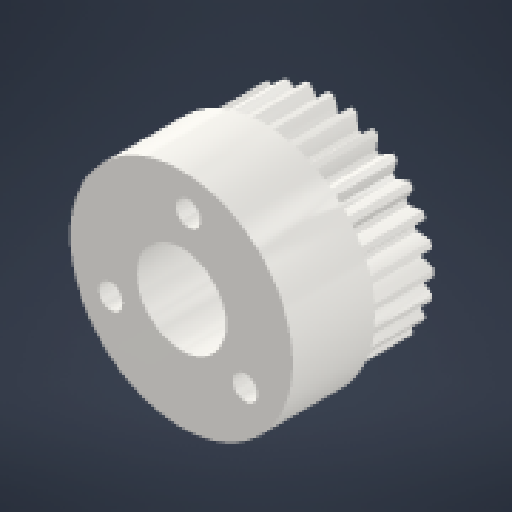
# Autodesk Inventor part: Spur Gear2
Saved by Autodesk Inventor 2025 (Build 290162000, 162)
## iProperties
CustomPartVersion: 1
Created: 2024-04-16
Part Number: Spur Gear2
Material: Steel
Document SubType Name: Modeling
Designer: sicia
Categories: <?xml version="1.0" encoding="UTF-16"?> <MemberInstance><Categories><FamilyTemplate><FamilyTemplateParameter ValueType="xs:double" Id="1" ObjectReferenceKey="da_z" ObjectType="kUserParameterObject"/><FamilyTemplateParameter ValueType="xs:double" Id="2" ObjectReferenceKey="da_b" ObjectType="kUserParameterObject"/><FamilyTemplateParameter ValueType="xs:double" Id="3" ObjectReferenceKey="da_beta" ObjectType="kUserParameterObject"/><FamilyTemplateParameter ValueType="xs:double" Id="4" ObjectReferenceKey="da_da" ObjectType="kUserParameterObject"/><FamilyTemplateParameter ValueType="xs:double" Id="5" ObjectReferenceKey="da_aw" ObjectType="kUserParameterObject"/><FamilyTemplateParameter ValueType="xs:string" Id="6" ObjectReferenceKey="EAIAABAAAACIAQAAAAAAAIAAAAAAAAAA" ObjectType="83910656" SubObjectId="SurfaceGeometry"/></FamilyTemplate><ParamToTemplateMap><ParamToTemplate CategoryParameter="//CategoryParameter[@InternalName='046C89C9-8512-4d59-83FE-43B91F4F132A']" TemplateParameter="1"/><ParamToTemplate CategoryParameter="//CategoryParameter[@InternalName='2552DF32-E462-4b46-AEBF-C6C7768E72AC']" TemplateParameter="2"/><ParamToTemplate CategoryParameter="//CategoryParameter[@InternalName='C9EE641D-15FC-4fae-A226-E94C4372FDD7']" TemplateParameter="3"/><ParamToTemplate><ParamToTemplate CategoryParameter="//CategoryParameter[@InternalName='00B6519A-459B-49c7-AD84-2E56D39A5744']" ConstantValue="0.770775"/></ParamToTemplate><ParamToTemplate><ParamToTemplate CategoryParameter="//CategoryParameter[@InternalName='04B31F0E-C7A6-4894-AA32-9629BEFACF47']" ConstantValue="1.000000"/></ParamToTemplate><ParamToTemplate><ParamToTemplate CategoryParameter="//CategoryParameter[@InternalName='43CBEC2E-7847-49e7-A936-2F7889FCB2D9']" ConstantValue="0.250000"/></ParamToTemplate><ParamToTemplate><ParamToTemplate CategoryParameter="//CategoryParameter[@InternalName='B1EFC894-105D-4ebd-86BF-FA20ED196853']" ConstantValue="0.333500"/></ParamToTemplate><ParamToTemplate><ParamToTemplate CategoryParameter="//CategoryParameter[@InternalName='51175063-3D10-4879-93E8-6246FE8B403D']" ConstantValue="2060000000.000000"/></ParamToTemplate><ParamToTemplate><ParamToTemplate CategoryParameter="//CategoryParameter[@InternalName='A3A52E27-4454-46a9-B0BD-C932399B70AF']" ConstantValue="0.300000"/></ParamToTemplate><ParamToTemplate><ParamToTemplate CategoryParameter="//CategoryParameter[@InternalName='91B76062-C214-41d9-B1B9-14D2AB99603D']" ConstantValue="0.150000"/></ParamToTemplate><ParamToTemplate><ParamToTemplate CategoryParameter="//CategoryParameter[@InternalName='374E806E-8B8A-4dda-A9AA-1039D6500AD2']" ConstantValue="6.666667"/></ParamToTemplate><ParamToTemplate><ParamToTemplate CategoryParameter="//CategoryParameter[@InternalName='2D373A89-B862-43d6-8D0B-0CBF12AB9F6C']" ConstantValue="0.349066"/></ParamToTemplate><ParamToTemplate CategoryParameter="//CategoryParameter[@InternalName='37777632-D6A2-4fac-9D53-DB8ACD95C989']" TemplateParameter="4"/><ParamToTemplate CategoryParameter="//CategoryParameter[@InternalName='FD1017F1-B727-4f7e-9707-0F86F1FF9423']" TemplateParameter="5"/><ParamToTemplate><ParamToTemplate CategoryParameter="//CategoryParameter[@InternalName='9E1B4470-B2D3-4ff1-B813-535BB4CDF51A']" ConstantValue="3520000.000000"/></ParamToTemplate><ParamToTemplate><ParamToTemplate CategoryParameter="//CategoryParameter[@InternalName='F8452263-BFF6-458c-9FB1-07C4B99E95CD']" ConstantValue="11400000.000000"/></ParamToTemplate><ParamToTemplate><ParamToTemplate CategoryParameter="//CategoryParameter[@InternalName='3E3BB259-FD49-497f-8171-6EBC954A3479']" ConstantValue="2.000000"/></ParamToTemplate><ParamToTemplate CategoryParameter="//CategoryParameter[@InternalName='27C3BAF2-7550-4e4b-AE2C-0DB134B7D9B7']" TemplateParameter="6"/></ParamToTemplateMap><Category DisplayName="Gear" InternalName="DC85795E-93AB-48d5-8EEE-5A27447B64BD" Mnemonic="Gear"><CategoryParameter DisplayName="z" InternalName="046C89C9-8512-4d59-83FE-43B91F4F132A" Mnemonic="z"/><CategoryParameter DisplayName="b" InternalName="2552DF32-E462-4b46-AEBF-C6C7768E72AC" Mnemonic="b"/><CategoryParameter DisplayName="||b|" InternalName="C9EE641D-15FC-4fae-A226-E94C4372FDD7" Mnemonic="beta"/><CategoryParameter DisplayName="x" InternalName="00B6519A-459B-49c7-AD84-2E56D39A5744" Mnemonic="x"/><CategoryParameter DisplayName="a*" InternalName="04B31F0E-C7A6-4894-AA32-9629BEFACF47" Mnemonic="a"/><CategoryParameter DisplayName="c*" InternalName="43CBEC2E-7847-49e7-A936-2F7889FCB2D9" Mnemonic="c"/><CategoryParameter DisplayName="r|.f|*" InternalName="B1EFC894-105D-4ebd-86BF-FA20ED196853" Mnemonic="rf"/><CategoryParameter DisplayName="E" InternalName="51175063-3D10-4879-93E8-6246FE8B403D" Mnemonic="E"/><CategoryParameter DisplayName="||m|" InternalName="A3A52E27-4454-46a9-B0BD-C932399B70AF" Mnemonic="mi"/><Category DisplayName="SpurGear" InternalName="26C5A22E-A91E-4dfd-A3B3-23CCAFAE1764" Mnemonic="SpurGear"><CategoryParameter DisplayName="m" InternalName="91B76062-C214-41d9-B1B9-14D2AB99603D" Mnemonic="m"/><CategoryParameter DisplayName="P" InternalName="374E806E-8B8A-4dda-A9AA-1039D6500AD2" Mnemonic="PP"/><CategoryParameter DisplayName="||a|" InternalName="2D373A89-B862-43d6-8D0B-0CBF12AB9F6C" Mnemonic="alpha"/><CategoryParameter DisplayName="d|.a|" InternalName="37777632-D6A2-4fac-9D53-DB8ACD95C989" Mnemonic="da"/><CategoryParameter DisplayName="a|.w|" InternalName="FD1017F1-B727-4f7e-9707-0F86F1FF9423" Mnemonic="aw"/><CategoryParameter DisplayName="||s||.Flim|" InternalName="9E1B4470-B2D3-4ff1-B813-535BB4CDF51A" Mnemonic="sFlim"/><CategoryParameter DisplayName="||s||.Hlim|" InternalName="F8452263-BFF6-458c-9FB1-07C4B99E95CD" Mnemonic="sHlim"/><CategoryParameter DisplayName="type" InternalName="3E3BB259-FD49-497f-8171-6EBC954A3479" Mnemonic="type"/><CategoryParameter DisplayName="PitchDiameter" InternalName="27C3BAF2-7550-4e4b-AE2C-0DB134B7D9B7" Mnemonic="IDS_PITCHDIAM"/></Category></Category></Categories></MemberInstance>
Density: 7.85 g/cm^3
Appearance: Steel
Mass: 368.86 g
Surface Area: 131.516 cm^2
Volume: 46.9885 cm^3
Author: sicia
Autodesk Inventor part; units mm, degrees
sketch "Sketch1" plane through (0, 0, 0) normal (0, 0, 1) x (1, 0, 0)
  circle A0 centre (0, 0) radius 23.3443
  dimension "d0" = 46.6886
  constraints: 1 centre point
  measures "d0" diameter of A0
extrude "Extrusion1" add sketch "Sketch1" along normal blind 10
ref_plane "Work Plane2" through (0, 0, 5) normal (0, 0, 1) x (1, 0, 0)
sketch "Sketch2" plane through (0, 0, 0) normal (0, 0, -1) x (-1, 0, 0)
  circle A0 centre (0, 0) radius 23.3443 projected
  circle A1 centre (0, 0) radius 21
  dimension "d3" = 42
  constraints: 1 centre point, 1 coincident
  measures "d3" diameter of A1
surface extrude "Pitch Diameter" sketch "Sketch2" against normal through all shown no curves A1
ref_plane "Work Plane8" through (0, 0, 0) normal (0.9937122, 0.1119645, 0) x (0, 0, 1)
ref_plane "Work Plane9" through (0, 0, 0) normal (1, 0, 0) x (0, 1, 0)
spur gear teeth "Spur Gear" teeth 28 pitch diameter 42 tip diameter 46.6886 root diameter 40.5623 face width 10 start plane through (0, 0, 0) normal (0, 0, -1) x (-1, 0, 0)
sketch "Sketch3" plane through (0, 0, 10) normal (0, 0, 1) x (1, 0, 0)
  arc A0 (-5.8309, 22.6044) -> (-6.1589, 19.3234) centre (6.5782, 19.7067) ccw projected
  arc A1 (-6.1589, 19.3234) -> (-7.2327, 18.9477) centre (0, 0) ccw projected
  arc A2 (-7.2327, 18.9477) -> (-9.5348, 21.3083) centre (-17.43, 11.3058) ccw projected
  arc A3 (-9.5348, 21.3083) -> (-10.7146, 20.7401) centre (0, 0) ccw projected
  arc A4 (-10.7146, 20.7401) -> (-10.3044, 17.4684) centre (2.0281, 20.6764) ccw projected
  arc A5 (-10.3044, 17.4684) -> (-11.2676, 16.8632) centre (0, 0) ccw projected
  arc A6 (-11.2676, 16.8632) -> (-14.0373, 18.6523) centre (-19.5088, 7.1439) ccw projected
  arc A7 (-14.0373, 18.6523) -> (-15.0611, 17.8359) centre (0, 0) ccw projected
  arc A8 (-15.0611, 17.8359) -> (-13.9331, 14.7375) centre (-2.6236, 20.6093) ccw projected
  arc A9 (-13.9331, 14.7375) -> (-14.7375, 13.9331) centre (0, 0) ccw projected
  arc A10 (-14.7375, 13.9331) -> (-17.8359, 15.0611) centre (-20.6093, 2.6236) ccw projected
  arc A11 (-17.8359, 15.0611) -> (-18.6523, 14.0373) centre (0, 0) ccw projected
  arc A12 (-18.6523, 14.0373) -> (-16.8632, 11.2676) centre (-7.1439, 19.5088) ccw projected
  arc A13 (-16.8632, 11.2676) -> (-17.4684, 10.3044) centre (0, 0) ccw projected
  arc A14 (-17.4684, 10.3044) -> (-20.7401, 10.7146) centre (-20.6764, -2.0281) ccw projected
  arc A15 (-20.7401, 10.7146) -> (-21.3083, 9.5348) centre (0, 0) ccw projected
  arc A16 (-21.3083, 9.5348) -> (-18.9477, 7.2327) centre (-11.3058, 17.43) ccw projected
  arc A17 (-18.9477, 7.2327) -> (-19.3234, 6.1589) centre (0, 0) ccw projected
  arc A18 (-19.3234, 6.1589) -> (-22.6044, 5.8309) centre (-19.7067, -6.5782) ccw projected
  arc A19 (-22.6044, 5.8309) -> (-22.8957, 4.5542) centre (0, 0) ccw projected
  arc A20 (-22.8957, 4.5542) -> (-20.082, 2.8351) centre (-14.9009, 14.4772) ccw projected
  arc A21 (-20.082, 2.8351) -> (-20.2094, 1.7046) centre (0, 0) ccw projected
  arc A22 (-20.2094, 1.7046) -> (-23.3351, 0.6547) centre (-17.7488, -10.7984) ccw projected
  arc A23 (-23.3351, 0.6547) -> (-23.3351, -0.6547) centre (0, 0) ccw projected
  arc A24 (-23.3351, -0.6547) -> (-20.2094, -1.7046) centre (-17.7488, 10.7984) ccw projected
  arc A25 (-20.2094, -1.7046) -> (-20.082, -2.8351) centre (0, 0) ccw projected
  arc A26 (-20.082, -2.8351) -> (-22.8957, -4.5542) centre (-14.9009, -14.4772) ccw projected
  arc A27 (-22.8957, -4.5542) -> (-22.6044, -5.8309) centre (0, 0) ccw projected
  arc A28 (-22.6044, -5.8309) -> (-19.3234, -6.1589) centre (-19.7067, 6.5782) ccw projected
  arc A29 (-19.3234, -6.1589) -> (-18.9477, -7.2327) centre (0, 0) ccw projected
  arc A30 (-18.9477, -7.2327) -> (-21.3083, -9.5348) centre (-11.3058, -17.43) ccw projected
  arc A31 (-21.3083, -9.5348) -> (-20.7401, -10.7146) centre (0, 0) ccw projected
  arc A32 (-20.7401, -10.7146) -> (-17.4684, -10.3044) centre (-20.6764, 2.0281) ccw projected
  arc A33 (-17.4684, -10.3044) -> (-16.8632, -11.2676) centre (0, 0) ccw projected
  arc A34 (-16.8632, -11.2676) -> (-18.6523, -14.0373) centre (-7.1439, -19.5088) ccw projected
  arc A35 (-18.6523, -14.0373) -> (-17.8359, -15.0611) centre (0, 0) ccw projected
  arc A36 (-17.8359, -15.0611) -> (-14.7375, -13.9331) centre (-20.6093, -2.6236) ccw projected
  arc A37 (-14.7375, -13.9331) -> (-13.9331, -14.7375) centre (0, 0) ccw projected
  arc A38 (-13.9331, -14.7375) -> (-15.0611, -17.8359) centre (-2.6236, -20.6093) ccw projected
  arc A39 (-15.0611, -17.8359) -> (-14.0373, -18.6523) centre (0, 0) ccw projected
  arc A40 (-14.0373, -18.6523) -> (-11.2676, -16.8632) centre (-19.5088, -7.1439) ccw projected
  arc A41 (-11.2676, -16.8632) -> (-10.3044, -17.4684) centre (0, 0) ccw projected
  arc A42 (-10.3044, -17.4684) -> (-10.7146, -20.7401) centre (2.0281, -20.6764) ccw projected
  arc A43 (-10.7146, -20.7401) -> (-9.5348, -21.3083) centre (0, 0) ccw projected
  arc A44 (-9.5348, -21.3083) -> (-7.2327, -18.9477) centre (-17.43, -11.3058) ccw projected
  arc A45 (-7.2327, -18.9477) -> (-6.1589, -19.3234) centre (0, 0) ccw projected
  arc A46 (-6.1589, -19.3234) -> (-5.8309, -22.6044) centre (6.5782, -19.7067) ccw projected
  arc A47 (-5.8309, -22.6044) -> (-4.5542, -22.8957) centre (0, 0) ccw projected
  arc A48 (-4.5542, -22.8957) -> (-2.8351, -20.082) centre (-14.4772, -14.9009) ccw projected
  arc A49 (-2.8351, -20.082) -> (-1.7046, -20.2094) centre (0, 0) ccw projected
  arc A50 (-1.7046, -20.2094) -> (-0.6547, -23.3351) centre (10.7984, -17.7488) ccw projected
  arc A51 (-0.6547, -23.3351) -> (0.6547, -23.3351) centre (0, 0) ccw projected
  arc A52 (0.6547, -23.3351) -> (1.7046, -20.2094) centre (-10.7984, -17.7488) ccw projected
  arc A53 (1.7046, -20.2094) -> (2.8351, -20.082) centre (0, 0) ccw projected
  arc A54 (2.8351, -20.082) -> (4.5542, -22.8957) centre (14.4772, -14.9009) ccw projected
  arc A55 (4.5542, -22.8957) -> (5.8309, -22.6044) centre (0, 0) ccw projected
  arc A56 (5.8309, -22.6044) -> (6.1589, -19.3234) centre (-6.5782, -19.7067) ccw projected
  arc A57 (6.1589, -19.3234) -> (7.2327, -18.9477) centre (0, 0) ccw projected
  arc A58 (7.2327, -18.9477) -> (9.5348, -21.3083) centre (17.43, -11.3058) ccw projected
  arc A59 (9.5348, -21.3083) -> (10.7146, -20.7401) centre (0, 0) ccw projected
  arc A60 (10.7146, -20.7401) -> (10.3044, -17.4684) centre (-2.0281, -20.6764) ccw projected
  arc A61 (10.3044, -17.4684) -> (11.2676, -16.8632) centre (0, 0) ccw projected
  arc A62 (11.2676, -16.8632) -> (14.0373, -18.6523) centre (19.5088, -7.1439) ccw projected
  arc A63 (14.0373, -18.6523) -> (15.0611, -17.8359) centre (0, 0) ccw projected
  arc A64 (15.0611, -17.8359) -> (13.9331, -14.7375) centre (2.6236, -20.6093) ccw projected
  arc A65 (13.9331, -14.7375) -> (14.7375, -13.9331) centre (0, 0) ccw projected
  arc A66 (14.7375, -13.9331) -> (17.8359, -15.0611) centre (20.6093, -2.6236) ccw projected
  arc A67 (17.8359, -15.0611) -> (18.6523, -14.0373) centre (0, 0) ccw projected
  arc A68 (18.6523, -14.0373) -> (16.8632, -11.2676) centre (7.1439, -19.5088) ccw projected
  arc A69 (16.8632, -11.2676) -> (17.4684, -10.3044) centre (0, 0) ccw projected
  arc A70 (17.4684, -10.3044) -> (20.7401, -10.7146) centre (20.6764, 2.0281) ccw projected
  arc A71 (20.7401, -10.7146) -> (21.3083, -9.5348) centre (0, 0) ccw projected
  arc A72 (21.3083, -9.5348) -> (18.9477, -7.2327) centre (11.3058, -17.43) ccw projected
  arc A73 (18.9477, -7.2327) -> (19.3234, -6.1589) centre (0, 0) ccw projected
  arc A74 (19.3234, -6.1589) -> (22.6044, -5.8309) centre (19.7067, 6.5782) ccw projected
  arc A75 (22.6044, -5.8309) -> (22.8957, -4.5542) centre (0, 0) ccw projected
  arc A76 (22.8957, -4.5542) -> (20.082, -2.8351) centre (14.9009, -14.4772) ccw projected
  arc A77 (20.082, -2.8351) -> (20.2094, -1.7046) centre (0, 0) ccw projected
  arc A78 (20.2094, -1.7046) -> (23.3351, -0.6547) centre (17.7488, 10.7984) ccw projected
  arc A79 (23.3351, -0.6547) -> (23.3351, 0.6547) centre (0, 0) ccw projected
  arc A80 (23.3351, 0.6547) -> (20.2094, 1.7046) centre (17.7488, -10.7984) ccw projected
  arc A81 (20.2094, 1.7046) -> (20.082, 2.8351) centre (0, 0) ccw projected
  arc A82 (20.082, 2.8351) -> (22.8957, 4.5542) centre (14.9009, 14.4772) ccw projected
  arc A83 (22.8957, 4.5542) -> (22.6044, 5.8309) centre (0, 0) ccw projected
  arc A84 (22.6044, 5.8309) -> (19.3234, 6.1589) centre (19.7067, -6.5782) ccw projected
  arc A85 (19.3234, 6.1589) -> (18.9477, 7.2327) centre (0, 0) ccw projected
  arc A86 (18.9477, 7.2327) -> (21.3083, 9.5348) centre (11.3058, 17.43) ccw projected
  arc A87 (21.3083, 9.5348) -> (20.7401, 10.7146) centre (0, 0) ccw projected
  arc A88 (20.7401, 10.7146) -> (17.4684, 10.3044) centre (20.6764, -2.0281) ccw projected
  arc A89 (17.4684, 10.3044) -> (16.8632, 11.2676) centre (0, 0) ccw projected
  arc A90 (16.8632, 11.2676) -> (18.6523, 14.0373) centre (7.1439, 19.5088) ccw projected
  arc A91 (18.6523, 14.0373) -> (17.8359, 15.0611) centre (0, 0) ccw projected
  arc A92 (17.8359, 15.0611) -> (14.7375, 13.9331) centre (20.6093, 2.6236) ccw projected
  arc A93 (14.7375, 13.9331) -> (13.9331, 14.7375) centre (0, 0) ccw projected
  arc A94 (13.9331, 14.7375) -> (15.0611, 17.8359) centre (2.6236, 20.6093) ccw projected
  arc A95 (15.0611, 17.8359) -> (14.0373, 18.6523) centre (0, 0) ccw projected
  arc A96 (14.0373, 18.6523) -> (11.2676, 16.8632) centre (19.5088, 7.1439) ccw projected
  arc A97 (11.2676, 16.8632) -> (10.3044, 17.4684) centre (0, 0) ccw projected
  arc A98 (10.3044, 17.4684) -> (10.7146, 20.7401) centre (-2.0281, 20.6764) ccw projected
  arc A99 (10.7146, 20.7401) -> (9.5348, 21.3083) centre (0, 0) ccw projected
  arc A100 (9.5348, 21.3083) -> (7.2327, 18.9477) centre (17.43, 11.3058) ccw projected
  arc A101 (7.2327, 18.9477) -> (6.1589, 19.3234) centre (0, 0) ccw projected
  arc A102 (6.1589, 19.3234) -> (5.8309, 22.6044) centre (-6.5782, 19.7067) ccw projected
  arc A103 (5.8309, 22.6044) -> (4.5542, 22.8957) centre (0, 0) ccw projected
  arc A104 (4.5542, 22.8957) -> (2.8351, 20.082) centre (14.4772, 14.9009) ccw projected
  arc A105 (2.8351, 20.082) -> (1.7046, 20.2094) centre (0, 0) ccw projected
  arc A106 (1.7046, 20.2094) -> (0.6547, 23.3351) centre (-10.7984, 17.7488) ccw projected
  arc A107 (0.6547, 23.3351) -> (-0.6547, 23.3351) centre (0, 0) ccw projected
  arc A108 (-0.6547, 23.3351) -> (-1.7046, 20.2094) centre (10.7984, 17.7488) ccw projected
  arc A109 (-1.7046, 20.2094) -> (-2.8351, 20.082) centre (0, 0) ccw projected
  arc A110 (-2.8351, 20.082) -> (-4.5542, 22.8957) centre (-14.4772, 14.9009) ccw projected
  arc A111 (-4.5542, 22.8957) -> (-5.8309, 22.6044) centre (0, 0) ccw projected
extrude "Extrusion2" add sketch "Sketch3" along normal blind 5
sketch "Sketch4" plane through (0, 0, 0) normal (0, 0, -1) x (-1, 0, 0)
  circle A0 centre (0, 0) radius 10
  dimension "d51" = 20
  constraints: 1 centre point, 1 coincident
  measures "d51" diameter of A0
sketch "Sketch5" plane through (0, 0, 15) normal (0, 0, 1) x (1, 0, 0)
  circle A0 centre (0, 0) radius 25
  dimension "d52" = 50
  constraints: 1 centre point, 1 coincident
  measures "d52" diameter of A0
ref_plane "Work Plane11" through (-108.543, -108.543, 33.5) normal (0, 0, -1) x (0.0880181, 0.9961189, 0)
extrude "Extrusion3" add sketch "Sketch5" along normal up to surface (18.5 mm away)
extrude "Extrusion4" cut sketch "Sketch4" against normal blind 33.5
sketch "Sketch6" plane through (0, 0, 33.5) normal (0, 0, 1) x (1, 0, 0)
  ellipse E0 centre (-17.2332, -3.035) end of major axis (-19.8176, -2.0941) minor radius 2.7503 projected
  ellipse E1 centre (11.2492, -13.4042) end of major axis (8.6656, -12.4636) minor radius 2.7495 projected
  ellipse E2 centre (5.9882, 16.4466) end of major axis (3.4046, 17.3872) minor radius 2.7494 projected
  point P0 (0, 0)
  constraints: 3 other
extrude "Extrusion5" cut sketch "Sketch6" against normal blind 20
equation "\"d0\" = da_da"
equation "\"d1\" = da_b"
equation "\"d3\" = da_d"
equation "\"d16\" = da_aw"
equation "\"d43\" = da_aw"
equation "\"d46\" = da_aw"
equation "\"da_da\" = 46.688563"
equation "\"da_b\" = 10"
equation "\"da_d\" = 42"
equation "\"da_aw\" = 44.000443"
body "Solid1"
body "Srf1"
